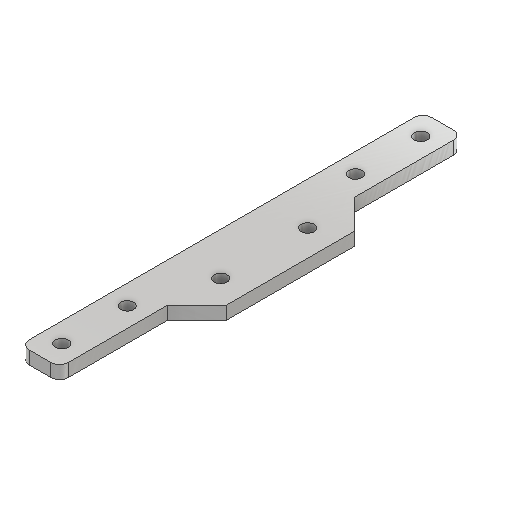
# Autodesk Inventor part: LC_ALU_3mm_X_Axis_Carriage_Accesory_Mounting_Bracket
Saved by Autodesk Inventor 2026.1 (Build 301233000, 233)
## iProperties
Created: 2016-06-18
Part Number: LC_ALU_3mm_X_Axis_Carriage_Accesory_Mounting_Bracket
Material: Ogólny
Document SubType Name: Modeling
Designer: Andrzej
Density: 1 g/cm^3
Appearance: Obrobione - aluminium
Mass: 3.17413 g
Surface Area: 27.8751 cm^2
Volume: 3.17413 cm^3
Author: Andrzej
Autodesk Inventor part; units mm, degrees
ref_plane "YZ Plane" through (0, 0, 0) normal (1, 0, 0) x (0, 1, 0)
ref_plane "XZ Plane" through (0, 0, 0) normal (0, 1, 0) x (-1, 0, 0)
ref_plane "XY Plane" through (0, 0, 0) normal (0, 0, 1) x (1, 0, 0)
sketch "Szkic1" plane through (0, 0, 0) normal (0, 0, 1) x (1, 0, 0)
  line L0 (0, 0) -> (15.75, 0)
  line L1 (15.75, 0) -> (15.75, 32.4)
  line L2 (0, 32.4) -> (15.75, 32.4)
  line L3 (0, 0) -> (0, 32.4)
  line L4 (0, 0) -> (9, 0)
  line L5 (9, 0) -> (9, -30)
  line L6 (9, -30) -> (0, -30)
  line L7 (0, -30) -> (0, 0)
  line L8 (0, 32.4) -> (9, 32.4)
  line L9 (9, 32.4) -> (9, 62.4)
  line L10 (9, 62.4) -> (0, 62.4)
  line L11 (0, 62.4) -> (0, 32.4)
  point P0 (15.1556, 0)
  point P1 (9.75, 26.2)
  point P2 (9.75, 6.2)
  point P3 (4.5, -25)
  point P4 (4.5, -10)
  point P5 (4.5, 42.4)
  point P6 (4.5, 57.4)
  dimension "d0" = 9.75
  dimension "d1" = 9.75
  dimension "d2" = 6.2
  dimension "d3" = 6.2
  dimension "d13" = 15.75
  dimension "d14" = 32.4
  dimension "d18" = 9
  dimension "d19" = 30
  dimension "d20" = 9
  dimension "d21" = 30
  dimension "d31" = 4.5
  dimension "d32" = 4.5
  dimension "d33" = 4.5
  dimension "d34" = 4.5
  dimension "d35" = 5
  dimension "d36" = 5
  dimension "d37" = 15
  dimension "d38" = 15
  constraints: 24 end point, 4 parallel, 2 horizontal, 2 perpendicular
  measures "d0" distance from line of point (9.75, 26.2) L3
  measures "d1" distance from line of L3 point (9.75, 6.2)
  measures "d2" distance from line of L2 point (9.75, 26.2)
  measures "d3" distance from line of L0 point (9.75, 6.2)
  measures "d13" distance of L0.start L0.end
  measures "d14" distance of L0.start L2.start
  measures "d18" distance of L5.end L6.end
  measures "d19" distance of L4.end L5.end
  measures "d20" distance of L10.end L9.end
  measures "d21" distance of L9.end L8.end
  measures "d31" distance from line of L7 point (4.5, -25)
  measures "d32" distance from line of L7 point (4.5, -10)
  measures "d33" distance from line of L11 point (4.5, 42.4)
  measures "d34" distance from line of L11 point (4.5, 57.4)
  measures "d35" distance from line of L6 point (4.5, -25)
  measures "d36" distance from line of L10 point (4.5, 57.4)
  measures "d37" distance of point (4.5, -25) point (4.5, -10)
  measures "d38" distance of point (4.5, 57.4) point (4.5, 42.4)
extrude "Wyciągnięcie proste1" add sketch "Szkic1" along normal blind 3 contours L3 L2 L1 L0
hole "Otwór1" at (9.75, 6.2, 0) at (9.75, 26.2, 0) direction (0, 0, 1) diameter 3 end through all
chamfer "Faza1" distance 1.5 angle 45 2 edges at (15.75, 0, 1.5) (15.75, 32.4, 1.5)
extrude "Wyciągnięcie proste2" add sketch "Szkic1" along normal blind 3 contours L0 L5 L6 L7 | L11 L10 L9 L2
chamfer "Faza2" distance 5.25 distance2 5.25 1 edges at (9, 32.4, 1.5) measured on face at (12.5, 32.4, 1)
chamfer "Faza3" distance 5.25 distance2 5.25 1 edges at (9, 0, 1.5) measured on face at (10.75, 0, 1)
fillet "Zaokrąglenie1" radius 2 4 edges at (9, -30, 1.5) (0, -30, 1.5) (9, 62.4, 1.5) (0, 62.4, 1.5)
hole "Otwór2" at (4.5, -25, 0) at (4.5, -10, 0) at (4.5, 42.4, 0) at (4.5, 57.4, 0) direction (0, 0, 1) diameter 3 end through all
equation "\"d1\" = d0"
equation "\"d3\" = d2"
equation "\"d18\" = d20"
equation "\"d19\" = d21"
equation "\"d35\" = d36"
